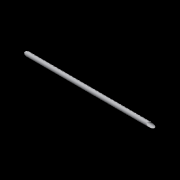
# Autodesk Inventor part: TuboEstructuraE
Saved by Autodesk Inventor 2016 (Build 200138000, 138)
## iProperties
Created: 2014-07-11
Part Number: TuboEstructuraE
Material: Steel, Galvanized
Document SubType Name: Modeling
Designer: Jose
Density: 7.85 g/cm^3
Appearance: Galvanized
Mass: 225.653 g
Surface Area: 575.854 cm^2
Volume: 28.7456 cm^3
Author: Jose
Autodesk Inventor part; units mm, degrees
ref_plane "YZ Plane" through (0, 0, 0) normal (1, 0, 0) x (0, 1, 0)
ref_plane "XZ Plane" through (0, 0, 0) normal (0, 1, 0) x (-1, 0, 0)
ref_plane "Work Plane1" through (605, -164.446, -59) normal (1, 0, 0) x (0, 1, 0)
sketch "Sketch1" plane through (0, 0, 0) normal (1, 0, 0) x (0, 1, 0)
  circle A0 centre (0, 0) radius 8
  circle A1 centre (0, 0) radius 7
  dimension "d0" = 16
  dimension "d1" = 1
  constraints: 2 centre point, 2 coincident
  measures "d0" diameter of A0
  measures "d1" radial gap between concentric circles of A0 A1
extrude "Extrusion1" add sketch "Sketch1" along normal blind 610
body "Solid1"
